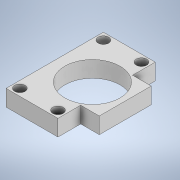
# Autodesk Inventor part: PodkladkaY
Saved by Autodesk Inventor 2020.1 (Build 241239000, 239)
## iProperties
Created: 2023-01-08
Part Number: PodkladkaY
Material: Типовые
Document SubType Name: Modeling
Designer: KirikDK
Density: 1 g/cm^3
Appearance: По умолчанию
Author: KirikDK
Autodesk Inventor part; units mm, degrees
ref_plane "YZ Plane" through (0, 0, 0) normal (1, 0, 0) x (0, 1, 0)
ref_plane "XZ Plane" through (0, 0, 0) normal (0, 1, 0) x (-1, 0, 0)
ref_plane "XY Plane" through (0, 0, 0) normal (0, 0, 1) x (1, 0, 0)
sketch "Эскиз1" plane through (0, 0, 0) normal (0, 1, 0) x (-1, 0, 0)
  circle A0 centre (-0.75, 2) radius 17
  line L0 (-5.25, -23.75) -> (-5.25, 27.75)
  line L1 (18.25, 27.75) -> (18.25, -23.75)
  line L2 (22.5, 32) -> (22.5, -28)
  line L3 (27.5, -33) -> (27.5, 37)
  circle A1 centre (18.25, -23.75) radius 3.25
  line L4 (18.25, -23.75) -> (-5.25, -23.75)
  arc A2 (16.5, -28) -> (22.5, -28) centre (19.5, -28) ccw
  line L5 (16.5, -28) -> (-3.5, -28)
  line L6 (-14.5, -33) -> (27.5, -33)
  circle A3 centre (-5.25, -23.75) radius 3.25
  arc A4 (-9.5, -28) -> (-3.5, -28) centre (-6.5, -28) ccw
  line L7 (-9.5, -28) -> (-9.5, -14)
  line L8 (-14.5, -19) -> (-14.5, -33)
  line L9 (-9.5, -14) -> (-21, -14)
  line L10 (-21, -14) -> (-21, -19)
  line L11 (-21, -19) -> (-14.5, -19)
  line L12 (-5.25, 27.75) -> (18.25, 27.75)
  circle A5 centre (18.25, 27.75) radius 3.25
  circle A6 centre (-5.25, 27.75) radius 3.25
  line L13 (-21, 18) -> (-9.5, 18)
  line L14 (-14.5, 23) -> (-21, 23)
  line L15 (-21, 23) -> (-21, 18)
  line L16 (-9.5, 18) -> (-9.5, 32)
  line L17 (-14.5, 37) -> (-14.5, 23)
  arc A7 (-3.5, 32) -> (-9.5, 32) centre (-6.5, 32) ccw
  line L18 (-3.5, 32) -> (16.5, 32)
  arc A8 (22.5, 32) -> (16.5, 32) centre (19.5, 32) ccw
  line L19 (27.5, 37) -> (-14.5, 37)
  line L20 (-21, 18) -> (-21, -14)
  line L21 (16.5, 32) -> (22.5, 32)
  line L22 (-3.5, 32) -> (-9.5, 32)
  line L23 (-3.5, -28) -> (-9.5, -28)
  line L24 (16.5, -28) -> (22.5, -28)
  point P0 (0, 0)
  point P1 (3.5, -18)
  dimension "d0" = 4.25
  dimension "d1" = 4.25
  dimension "d2" = 4.25
  dimension "d3" = 4.25
  dimension "d4" = 19
  dimension "d5" = 34
  constraints: 50 end point, 9 centre point, 8 point on circle, 4 coincident, 4 collinear, 3 parallel, 2 horizontal, 1 perpendicular, 1 vertical
  measures "d0" distance between parallel lines of L18 L12
  measures "d1" distance between parallel lines of L5 L4
  measures "d2" distance between parallel lines of L2 L1
  measures "d3" distance between parallel lines of L7 L0
  measures "d4" distance from line of L1 A0.centre
  measures "d5" diameter of A0
extrude "Выдавливание1" add sketch "Эскиз1" along normal blind 10 contours A0 L0 A6 L12 A5 L1 A1 L4 A3 | L2 L24 L5 L23 L7 L9 L20 L13 L16 L22 L18 L21
